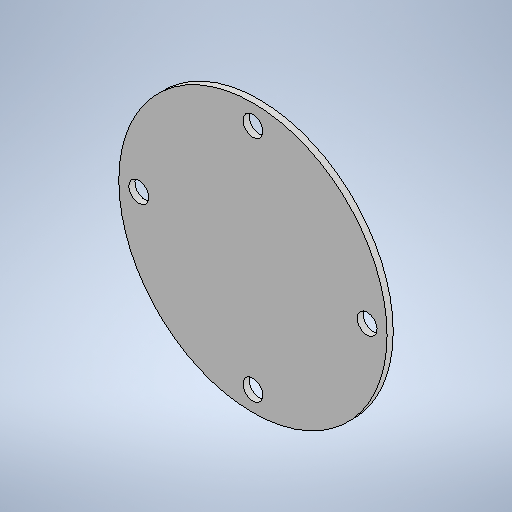
# Autodesk Inventor part: MSC 904 FLANGE BASE TUBE
Saved by Autodesk Inventor 2025 (Build 290162010, 162A)
## iProperties
Created: 2024-07-01
Part Number: MSC 904 FLANGE BASE TUBE
Material: Stainless Steel
Document SubType Name: Sheet Metal
Designer: pokla
Density: 8 g/cm^3
Sheet Metal Rule: AISI304 3mm Die 32
Appearance: Default
Stock Number: МОО 904 фланец базовой трубы
Mass: 755.214 g
Surface Area: 500.032 cm^2
Volume: 94.4017 cm^3
Flat Pattern Width: 17.5 cm
Flat Pattern Length: 17.5 cm
Flat Pattern Area: 306.25 cm^2
Sheet Metal Width: 175,000 mm
Sheet Metal Length: 175,000 mm
Sheet Metal Area: 30625,000 mm^2
Author: pokla
Autodesk Inventor part; units mm, degrees
ref_plane "YZ Plane" through (0, 0, 0) normal (1, 0, 0) x (0, 1, 0)
ref_plane "XZ Plane" through (0, 0, 0) normal (0, 1, 0) x (-1, 0, 0)
ref_plane "XY Plane" through (0, 0, 0) normal (0, 0, 1) x (1, 0, 0)
sketch "Sketch1" plane through (0, 0, 0) normal (0, 1, 0) x (-1, 0, 0)
  circle A0 centre (0, 0) radius 87.5
  dimension "d0" = 175
  measures "d0" diameter of A0
extrude "Plate1" add sketch "Sketch1" along normal blind 4
sketch "Sketch2" plane through (0, 4, 0) normal (0, 1, 0) x (1, 0, 0)
  line L0 (-40, -40) -> (40, -40) construction
  line L1 (40, -40) -> (40, 40) construction
  line L2 (40, 40) -> (-40, 40) construction
  line L3 (-40, 40) -> (-40, -40) construction
  line L4 (40, -40) -> (-40, 40) construction
  circle A0 centre (0, 0) radius 87.5 projected
  line L5 (0, 0) -> (0, -87.5) construction
  circle A1 centre (0, -74.5) radius 6.5
  dimension "d2" = 80
  dimension "d3" = 80
  dimension "d16" = 13
  dimension "d23" = 74.5
  constraints: 12 end point, 2 parallel, 2 perpendicular, 1 centre point, 1 coincident, 1 horizontal, 1 midpoint, 1 point on line, 1 vertical alignment, 1 other
  measures "d2" distance of L2.end L1.end
  measures "d3" distance of L1.end L0.end
  measures "d16" diameter of A1
  measures "d23" distance of A1.centre point (0, 0)
extrude "Extrusion1" cut sketch "Sketch2" against normal through all contours A1
pattern_circular "Circular Pattern1" count 4 over 360 about axis through (0, -10, 0) along (0, 1, 0) of "Extrusion1"
sketch "Sketch3" plane through (0, 4, 0) normal (0, 1, 0) x (1, 0, 0)
  line L0 (9.823, 55.7091) -> (-55.7091, 9.823)
  line L1 (-55.7091, 9.823) -> (-9.823, -55.7091)
  line L2 (-9.823, -55.7091) -> (55.7091, -9.823)
  line L3 (55.7091, -9.823) -> (9.823, 55.7091) construction
  line L4 (32.7661, 22.9431) -> (-32.7661, -22.9431) construction
  line L5 (0, 0) -> (26.1739, 0) construction
  line L6 (-55.7091, -9.823) -> (9.823, -55.7091)
  line L7 (9.823, -55.7091) -> (55.7091, 9.823)
  line L8 (55.7091, 9.823) -> (-9.823, 55.7091) construction
  line L9 (-9.823, 55.7091) -> (-55.7091, -9.823)
  line L10 (22.9431, 32.7661) -> (-22.9431, -32.7661)
  line L11 (9.823, -55.7091) -> (39.823, -55.7091)
  line L12 (-55.7091, 9.823) -> (-55.7091, 39.823)
  dimension "d18" = 80
  dimension "d19" = 35
  dimension "d20" = 55
  dimension "d21" = 30
  dimension "d22" = 30
  constraints: 26 end point, 6 midpoint, 4 parallel, 3 equal length, 2 horizontal, 2 perpendicular, 1 coincident, 1 vertical
  measures "d18" distance of L2.end L0.start
  measures "d19" angle of L4 L5
  measures "d20" angle of L5 L10
  measures "d21" distance of L6.end L11.end
  measures "d22" distance of L0.end L12.end
mark "Mark1"
equation "\"d1\" = Thickness"
equation "\"BendReliefWidth\" = Thickness"
equation "\"BendReliefDepth\" = 0.5 * Thickness"
equation "\"CornerReliefSize\" = 4 * Thickness"
equation "\"MinimumRemnant\" = 2 * Thickness"
equation "\"TransitionRadius\" = BendRadius"
equation "\"JacobiRadiusSize\" = BendRadius"
equation "\"GapSize\" = Thickness"
equation "\"Thickness\" = 4"
equation "\"BendRadius\" = 5"
body "Solid1"
